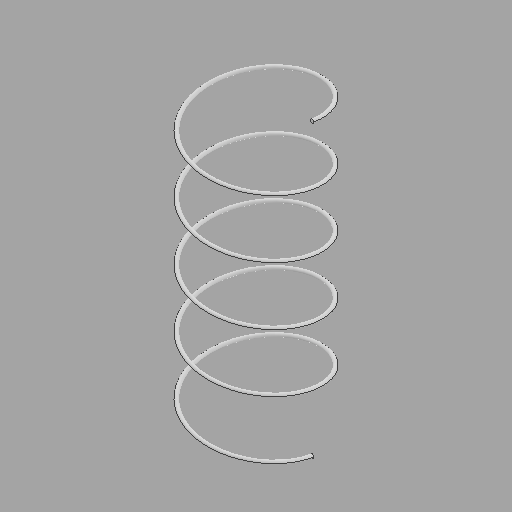
# Autodesk Inventor part: CE-9.3.1-01-002
Saved by Autodesk Inventor 2024 (Build 280153000, 153)
## iProperties
Created: 2024-03-22
Part Number: CE-9.3.1-01-002
Material: Generic
Document SubType Name: Modeling
Designer: Alex
Density: 1 g/cm^3
Appearance: Default
Author: Alex
Autodesk Inventor part; units mm, degrees
ref_plane "YZ Plane" through (0, 0, 0) normal (1, 0, 0) x (0, 1, 0)
ref_plane "XZ Plane" through (0, 0, 0) normal (0, 1, 0) x (-1, 0, 0)
ref_plane "XY Plane" through (0, 0, 0) normal (0, 0, 1) x (1, 0, 0)
sketch "Sketch1" plane through (0, 0, 0) normal (0, 0, 1) x (1, 0, 0)
  line L0 (40, 0) -> (-40, 0) projected
  line L1 (40, 200) -> (-40, 200) projected
  line L2 (0, 200) -> (0, 0)
  line L3 (-37.46, 200) -> (37.46, 200)
  dimension "d0" = 80
  dimension "d1" = 200
  dimension "d2" = 74.92
  constraints: 4 end point, 3 midpoint, 1 horizontal, 1 vertical
  measures "d0" distance of L1.start L1.end
  measures "d1" distance of L2.start L2.end
  measures "d2" distance of L3.start L3.end
sketch "Sketch2" plane through (0, 0, 0) normal (0, 0, 1) x (1, 0, 0)
  line L0 (40, 0) -> (-40, 0) construction
  circle A0 centre (38.73, 0) radius 1.27
  point P0 (0, 0)
  dimension "d3" = 2.54
  constraints: 1 horizontal alignment, 1 point on line, 2 other
coil "Coil1" sketch "Sketch2" operation add axis through (0, 200, 0) along (0, 1, 0) pitch 40 turns 5 hand left
equation "\"d5\" = d1"
body "Solid1"
